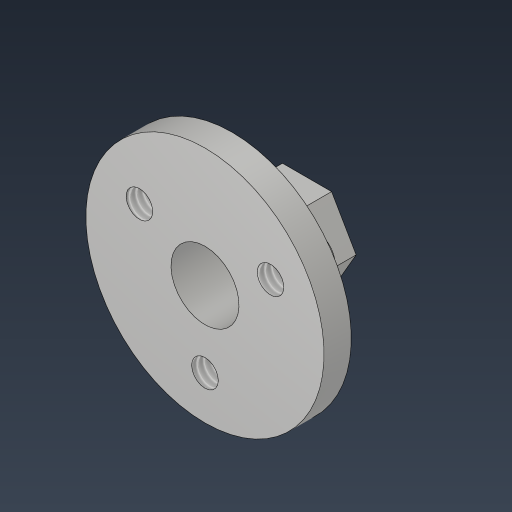
# Autodesk Inventor part: Encoder Klemmscheibe
Saved by Autodesk Inventor 2023.1 (Build 271208000, 208)
## iProperties
Part Number: Encoder Klemmscheibe
Material: Aluminium 6061
Document SubType Name: Modeling
Designer: rYan
Mass: 1.29779 g
Surface Area: 10.6814 cm^2
Volume: 0.480664 cm^3
Density: 2.7 g/cm^3
Appearance: Aluminium - flach
Author: rYan
Autodesk Inventor part; units mm, degrees
ref_plane "YZ Plane" through (0, 0, 0) normal (1, 0, 0) x (0, 1, 0)
ref_plane "XZ Plane" through (0, 0, 0) normal (0, 1, 0) x (-1, 0, 0)
ref_plane "XY Plane" through (0, 0, 0) normal (0, 0, 1) x (1, 0, 0)
sketch "Skizze3" plane through (0, 0, 0) normal (1, 0, 0) x (0, 1, 0)
  line L0 (9.15, 0) -> (0, 0)
  line L1 (1.6, 5.55) -> (2.7, 5.55)
  line L2 (2.7, 5.55) -> (2.7, 2)
  line L3 (2.7, 2) -> (0, 2)
  line L4 (0, 2) -> (0, 7)
  line L5 (0, 7) -> (1.6, 7)
  line L6 (1.6, 7) -> (1.6, 5.55)
  dimension "d17" = 4
  dimension "d18" = 11.1
  dimension "d24" = 14
  dimension "d69" = 1.6
  dimension "d75" = 1.1
  constraints: 14 end point, 3 perpendicular, 3 point on line, 1 horizontal
  measures "d17" diameter of L3 L0
  measures "d18" diameter of L1 L0
  measures "d24" diameter of L5 L0
  measures "d69" distance between parallel lines of L4 L6
  measures "d75" distance between parallel lines of L6 L2
sketch "Skizze3 outline for Umdrehung1" plane through (0, 0, 0) normal (1, 0, 0) x (0, 1, 0)
  line L0 (1.6, 7) -> (0, 7)
  line L1 (1.6, 5.55) -> (1.6, 7)
  line L2 (2.7, 5.55) -> (1.6, 5.55)
  line L3 (2.7, 2) -> (2.7, 5.55)
  line L4 (0, 2) -> (2.7, 2)
  line L5 (0, 7) -> (0, 2)
revolve "Umdrehung1" add sketch "Skizze3 outline for Umdrehung1" angle 360 about axis through (0, 9.15, 0) along (0, -1, 0)
sketch "Skizze8" plane through (0, 2.7, 0) normal (0, 1, 0) x (1, 0, 0)
  circle A0 centre (0, 0) radius 5.55
  arc A1 (0.760995, -4.975916) -> (1.898212, -5.215294) centre (1.52199, -4.181632) ccw
  arc A2 (0.760995, -4.975916) -> (-0.760995, -4.975916) centre (0, -5.7702) ccw
  arc A3 (-1.898212, -5.215294) -> (-0.760995, -4.975916) centre (-1.52199, -4.181632) ccw
  line L0 (0, 9.8) -> (0, -9.8) construction
  line L1 (-1.898212, -5.215294) -> (0, 0) construction
  dimension "d59" = 1.1
  dimension "d60" = 1.1
  dimension "d61" = 20
  constraints: 8 point on circle, 4 tangent, 3 centre point, 2 end point, 1 other
  measures "d59" radius of A1
  measures "d60" radius of A2
  measures "d61" angle of L1 L0
sketch "Skizze8 outline for Extrusion5" plane through (0, 2.7, 0) normal (0, 1, 0) x (1, 0, 0)
  arc A0 (0.760995, -4.975916) -> (-0.760995, -4.975916) centre (0, -5.7702) ccw
  arc A1 (1.898212, -5.215294) -> (0.760995, -4.975916) centre (1.52199, -4.181632) cw
  arc A2 (-1.898212, -5.215294) -> (1.898212, -5.215294) centre (0, 0) ccw
  arc A3 (-0.760995, -4.975916) -> (-1.898212, -5.215294) centre (-1.52199, -4.181632) cw
extrude "Extrusion5" cut sketch "Skizze8 outline for Extrusion5" against normal up to surface (1.1 mm away)
pattern_circular "Runde Anordnung2" count 9 over 360 about axis through (0, -10, 0) along (0, 1, 0) of "Extrusion5"
sketch "Skizze9" plane through (0, 2.7, 5.7702) normal (0, 1, 0) x (1, 0, 0)
  circle A0 centre (0, 5.7702) radius 3 construction
  line L0 (0, 15.5702) -> (0, -4.0298) construction
  circle A1 centre (0, 5.7702) radius 2
  line L1 (-1.443376, 3.2702) -> (-2.886751, 5.7702)
  line L2 (-2.886751, 5.7702) -> (-1.443376, 8.2702)
  line L3 (-1.443376, 8.2702) -> (1.443376, 8.2702)
  line L4 (1.443376, 8.2702) -> (2.886751, 5.7702)
  line L5 (2.886751, 5.7702) -> (1.443376, 3.2702)
  line L6 (1.443376, 3.2702) -> (-1.443376, 3.2702)
  circle A2 centre (0, 10.2202) radius 1 construction
  arc A3 (0.986762, 10.706307) -> (-0.986762, 10.706307) centre (0, 10.2202) ccw construction
  line L7 (1.443376, 3.2702) -> (0, 5.7702)
  line L8 (0, 5.7702) -> (-1.443376, 3.2702)
  line L9 (1, 4.038149) -> (1, 3.2702)
  line L10 (-1, 4.038149) -> (-1, 3.2702)
  line L11 (1.443376, 3.2702) -> (1.443376, 4.385763)
  line L12 (-1.443376, 3.2702) -> (-1.443376, 4.385763)
  point P0 (0, 7.7702)
  point P1 (0, 11.2202)
  point P2 (1, 4.038149)
  point P3 (-1, 4.038149)
  dimension "d92" = 2
  dimension "d70" = 6
  dimension "d74" = 4
  dimension "d89" = 0.5
  dimension "d90" = 5
  dimension "d91" = 4.45
  constraints: 24 end point, 6 point on line, 5 point on circle, 3 coincident, 3 parallel, 1 centre point, 1 horizontal, 1 perpendicular, 1 vertical alignment, 15 other
  measures "d70" diameter of A0
  measures "d74" diameter of A1
  measures "d89" distance from line of L3 A1.start
  measures "d90" distance between parallel lines of L3 L6
  measures "d91" distance of point (0, 10.22) point (0, 5.77)
sketch "Skizze9 outline for Extrusion6" plane through (0, 2.7, 5.7702) normal (0, 1, 0) x (1, 0, 0)
  circle A0 centre (0, 5.7702) radius 2
  line L0 (1.443376, 3.2702) -> (2.886751, 5.7702)
  line L1 (2.886751, 5.7702) -> (1.443376, 8.2702)
  line L2 (1.443376, 8.2702) -> (-1.443376, 8.2702)
  line L3 (-1.443376, 8.2702) -> (-2.886751, 5.7702)
  line L4 (-2.886751, 5.7702) -> (-1.443376, 3.2702)
  line L5 (-1.443376, 3.2702) -> (1.443376, 3.2702)
extrude "Extrusion6" add sketch "Skizze9 outline for Extrusion6" along normal blind 3.3
hole "Bohrung3" at (0, 2.7, -4.45) direction (0, -1, 0) diameter 1.567 end through all thread size "M2x0.4" class "6H" standard "ISO Metric profile"
pattern_circular "Runde Anordnung3" count 3 over 360 about axis through (0, -10, 0) along (0, 1, 0) of "Bohrung3", "Extrusion6"
